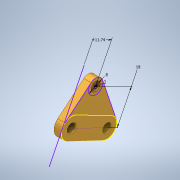
# Autodesk Inventor part: Kauri modular camera mount nano cam
Saved by Autodesk Inventor 2020 (Build 240168000, 168)
## iProperties
Created: 2022-05-05
Part Number: Kauri modular camera mount nano cam
Material: Brass, Soft Yellow
Document SubType Name: Modeling
Designer: Steven
Density: 8.47 g/cm^3
Appearance: Brass - Satin
Mass: 18.7081 g
Surface Area: 16.7722 cm^2
Volume: 2.20875 cm^3
Author: Steven
Autodesk Inventor part; units mm, degrees
ref_plane "YZ Plane" through (0, 0, 0) normal (1, 0, 0) x (0, 1, 0)
ref_plane "XZ Plane" through (0, 0, 0) normal (0, 1, 0) x (-1, 0, 0)
ref_plane "XY Plane" through (0, 0, 0) normal (0, 0, 1) x (1, 0, 0)
sketch "Sketch1" plane through (0, 0, 0) normal (1, 0, 0) x (0, 1, 0)
  circle A0 centre (-9.7574, -19.7073) radius 1.55 construction
  circle A1 centre (0, 0) radius 1.55 construction
  circle A2 centre (-9.7574, -19.7073) radius 2.55
  circle A3 centre (0, 0) radius 2.55
  line L0 (-6.0684, -24.2876) -> (12.7398, 12.1607) construction
  arc A4 (-12.2239, -24.4871) -> (-4.9776, -22.1738) centre (-9.7574, -19.7073) ccw
  circle A5 centre (0, 0) radius 5.7448
  line L1 (-4.9776, -22.1738) -> (5.1052, -2.6344)
  arc A6 (-4.9776, -22.1738) -> (-12.2239, -24.4871) centre (-9.7574, -19.7073) ccw
  line L2 (-14.5372, -17.2408) -> (-5.1904, 2.4623)
  line L3 (0, 0) -> (0, -27.0135) construction
  line L4 (0, 0) -> (-9.7574, -19.7073) construction
  point P0 (-10.1101, -25.5779)
  dimension "d0" = 5.1
  dimension "d1" = 5.1
  dimension "d3" = 11.4897
  dimension "d4" = 5.3787
  dimension "d5" = 21.8076
  dimension "d6" = 21.9875
  constraints: 10 end point, 7 centre point, 7 point on circle, 4 coincident, 2 tangent, 1 point on line, 1 vertical
  measures "d0" diameter of A2
  measures "d1" diameter of A3
  measures "d3" diameter of A5
  measures "d4" radius of A6
  measures "d5" distance of L2.start L2.end
  measures "d6" distance of L1.start L1.end
extrude "Extrusion1" add sketch "Sketch1" along normal blind 4
sketch "Sketch2" plane through (4, 0, 0) normal (1, 0, 0) x (0, 0, -1)
  arc A0 (17.2408, -14.5372) -> (22.1738, -4.9776) centre (19.7073, -9.7574) ccw projected
  line L0 (22.1738, -4.9776) -> (2.6344, 5.1052) projected
  arc A1 (2.6344, 5.1052) -> (-2.4623, -5.1904) centre (0, 0) ccw projected
  line L1 (-2.4623, -5.1904) -> (17.2408, -14.5372) construction
  circle A2 centre (19.7073, -9.7574) radius 2.55 construction
  circle A3 centre (0, 0) radius 2.55 construction
  circle A4 centre (19.7073, -9.7574) radius 2.55 construction
  line L2 (-0.0042, 0.0021) -> (19.7073, -9.7574) construction
  circle A5 centre (13.3596, 13.4709) radius 1
  circle A6 centre (13.3596, 13.4709) radius 4
  line L3 (10.7905, 16.5368) -> (-3.6897, 4.4033)
  arc A7 (2.6344, 5.1052) -> (-2.4623, -5.1904) centre (0, 0) ccw projected
  line L4 (17.1514, 14.7445) -> (24.806, -8.0448)
  line L5 (-12.5084, -12.3162) -> (6.9664, 27.0174)
  point P0 (-3.6897, 4.4033)
  dimension "d11" = 2
  dimension "d12" = 8
  dimension "d20" = 18
  dimension "d21" = 11.7401
  constraints: 8 end point, 5 tangent, 4 point on circle, 2 centre point, 1 coincident, 1 perpendicular
  measures "d11" diameter of A5
  measures "d12" diameter of A6
  measures "d20" distance from line of L2 A5.centre
  measures "d21" distance from line of A5.centre L5
extrude "Extrusion2" add sketch "Sketch2" against normal up to surface (4 mm away)
sketch "Sketch3" plane through (4, 0, 0) normal (1, 0, 0) x (0, 0, -1)
  circle A0 centre (13.3596, 13.4709) radius 1 projected
  circle A1 centre (13.3596, 13.4709) radius 2.5
  point P0 (0, 0)
  dimension "d15" = 5
  constraints: 1 centre point, 1 coincident
  measures "d15" diameter of A1
extrude "Extrusion3" cut sketch "Sketch3" against normal blind 2
body "Solid1"
